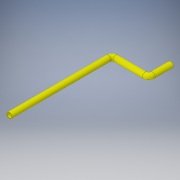
# Autodesk Inventor part: ABS Arm
Saved by Autodesk Inventor 2016 (Build 200138000, 138)
## iProperties
Created: 2015-07-12
Part Number: ABS Arm
Material: ABS Plastic
Document SubType Name: Modeling
Designer: steele
Density: 1.06 g/cm^3
Appearance: Smooth - Yellow
Author: steele
Autodesk Inventor part; units mm, degrees
ref_plane "YZ Plane" through (0, 0, 0) normal (1, 0, 0) x (0, 1, 0)
ref_plane "XZ Plane" through (0, 0, 0) normal (0, 1, 0) x (-1, 0, 0)
ref_plane "XY Plane" through (0, 0, 0) normal (0, 0, 1) x (1, 0, 0)
sketch "Sketch1" plane through (0, 0, 0) normal (0, 1, 0) x (-1, 0, 0)
  line L0 (0, 0) -> (0, 63.5)
  line L1 (12.7, 76.2) -> (114.3, 76.2)
  line L2 (127, 88.9) -> (127, 431.8)
  arc A0 (114.3, 76.2) -> (127, 88.9) centre (114.3, 88.9) ccw
  arc A1 (12.7, 76.2) -> (0, 63.5) centre (12.7, 63.5) ccw
  point P0 (0, 76.2)
  point P1 (127, 76.2)
  dimension "short" = 76.2
  dimension "right" = 127
  dimension "long" = 355.6
  dimension "turn_radisu" = 12.7
  dimension "d10" = 12.7
  constraints: 6 end point, 4 point on circle, 4 point on line, 4 tangent, 2 centre point, 2 perpendicular, 1 vertical
  measures "short" distance of L0.start point (0, 76.2)
  measures "right" distance of point (0, 76.2) point (127, 76.2)
  measures "long" distance of point (127, 76.2) L2.end
  measures "turn_radisu" radius of A0
  measures "d10" radius of A1
sketch "Sketch2" plane through (0, 0, 0) normal (0, 0, 1) x (1, 0, 0)
  circle A0 centre (0, 0) radius 9.525
  circle A1 centre (0, 0) radius 7.62
  dimension "outside_diamter" = 19.05
  dimension "inside_diameter" = 15.24
  constraints: 2 centre point, 2 coincident
  measures "outside_diamter" diameter of A0
  measures "inside_diameter" diameter of A1
sweep "Sweep2" add profiles "Sketch2" path "Sketch1" path curves L0 A1 L1 A0 L2
body "Solid2"
